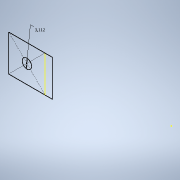
# Autodesk Inventor part: 13_Motor_Fixation_Thread_Mount
Saved by Autodesk Inventor 2021 (Build 250183000, 183)
## iProperties
Created: 2021-08-05
Part Number: 13_Motor_Fixation_Thread_Mount
Material: Generisch
Document SubType Name: Modeling
Designer: User
Density: 1 g/cm^3
Appearance: Vorgabe
Author: User
Autodesk Inventor part; units mm, degrees
ref_plane "YZ Plane" through (0, 0, 0) normal (1, 0, 0) x (0, 1, 0)
ref_plane "XZ Plane" through (0, 0, 0) normal (0, 1, 0) x (-1, 0, 0)
ref_plane "XY Plane" through (0, 0, 0) normal (0, 0, 1) x (1, 0, 0)
sketch "Skizze1" plane through (0, 0, 0) normal (0, 0, 1) x (1, 0, 0)
  line L0 (-41.8, 0) -> (-41.8, -12) projected
  line L1 (-53.8, -12) -> (-41.8, -12) projected
  line L2 (-53.8, 0) -> (-53.8, -12) projected
  line L3 (-41.8, 0) -> (-53.8, 0) projected
  line L4 (-39.4, 0) -> (-39.4, -12) projected
  line L5 (-41.8, -12) -> (-53.8, 0) construction
  line L6 (-53.8, -12) -> (-41.8, 0) construction
  circle A0 centre (-47.8, -6) radius 1.675
  line L7 (-39.4, -12) -> (-53.8, -12)
  line L8 (-53.8, -12) -> (-53.8, 0)
  line L9 (-53.8, 0) -> (-39.4, 0)
  line L10 (-39.4, 0) -> (-39.4, -12)
  point P0 (0, 0)
  dimension "d0" = 3.35
  constraints: 12 end point, 2 parallel, 2 perpendicular, 1 centre point, 1 horizontal, 1 midpoint
  measures "d0" diameter of A0
extrude "Extrusion1" add sketch "Skizze1" along normal blind 6
